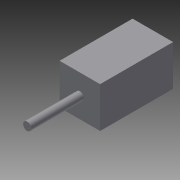
# Autodesk Inventor part: horrible gearbox
Saved by Autodesk Inventor 2013 (Build 170138000, 138)
## iProperties
Created: 2013-01-31
Part Number: horrible gearbox
Material: Generic
Document SubType Name: Modeling
Designer: Arpan
Density: 1 g/cm^3
Author: Arpan
Autodesk Inventor part; units mm, degrees
ref_plane "YZ Plane" through (0, 0, 0) normal (1, 0, 0) x (0, 1, 0)
ref_plane "XZ Plane" through (0, 0, 0) normal (0, 1, 0) x (-1, 0, 0)
ref_plane "XY Plane" through (0, 0, 0) normal (0, 0, 1) x (1, 0, 0)
sketch "Sketch1" plane through (0, 0, 0) normal (0, 0, 1) x (1, 0, 0)
  line L0 (0, 0) -> (-63.5, 0)
  line L1 (-63.5, 0) -> (-63.5, 63.5)
  line L2 (-63.5, 63.5) -> (0, 63.5)
  line L3 (0, 63.5) -> (0, 0)
  dimension "d0" = 63.5
  dimension "d1" = 63.5
  constraints: 8 end point, 2 perpendicular, 1 horizontal, 1 parallel
  measures "d0" distance of L0.start L0.end
  measures "d1" distance of L0.end L1.end
extrude "Extrusion1" add sketch "Sketch1" along normal blind 114.4016
sketch "Sketch2" plane through (0, 0, 114.4016) normal (0, 0, 1) x (1, 0, 0)
  line L0 (-63.5, 63.5) -> (-63.5, 0) projected
  line L1 (-63.5, 31.75) -> (-31.75, 31.75)
  circle A0 centre (-31.75, 31.75) radius 6.35
  dimension "d4" = 12.7
  constraints: 2 end point, 1 centre point, 1 coincident, 1 midpoint, 1 perpendicular
  measures "d4" diameter of A0
extrude "Extrusion2" add sketch "Sketch2" along normal blind 82.55
body "Solid1"
